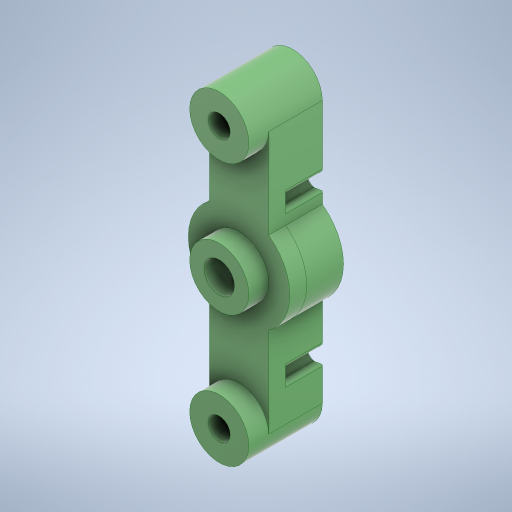
# Autodesk Inventor part: DualPMTController.MidSpacer
Saved by Autodesk Inventor 2023 (Build 270158000, 158)
## iProperties
Created: 2023-09-26
Part Number: DualPMTController.MidSpacer
Material: Generic
Document SubType Name: Modeling
Designer: Graeme
Density: 1 g/cm^3
Appearance: Default
Mass: 1.63627 g
Surface Area: 17.3966 cm^2
Volume: 1.63627 cm^3
Author: Graeme
Autodesk Inventor part; units mm, degrees
sketch "Sketch1" plane through (0, 0, 0) normal (0, 0, 1) x (1, 0, 0)
  circle A0 centre (0, 15.5) radius 1.55 projected
  circle A1 centre (0, 15.5) radius 3.5
  circle A2 centre (0, -15.5) radius 1.55 projected
  circle A3 centre (0, -15.5) radius 3.5
  circle A4 centre (0, 15.5) radius 1.3
  circle A5 centre (0, -15.5) radius 1.3
  point P0 (0, 0)
  dimension "d0" = 7
  dimension "d1" = 7
  dimension "d29" = 2.6
  dimension "d30" = 2.6
  constraints: 4 centre point, 4 coincident
  measures "d0" diameter of A1
  measures "d1" diameter of A3
  measures "d29" diameter of A4
  measures "d30" diameter of A5
ref_plane "Work Plane1" through (-88.8, 12.7, 8.6873) normal (0, 0, 1) x (1, 0, 0)
extrude "Extrusion1" add sketch "Sketch1" along normal up to surface (8.6873 mm away) contours A0 | A1 | A2 | A3
ref_plane "Work Plane2" through (0, 15.5, 4.3437) normal (0, 0, 1) x (1, 0, 0)
sketch "Sketch2" plane through (0, 15.5, 4.3437) normal (0, 0, 1) x (1, 0, 0)
  circle A0 centre (0, 0) radius 3.5 projected
  circle A1 centre (0, -31) radius 3.5 projected
  line L0 (3, -18.2) -> (3, -16.5) projected
  line L1 (3, -16.5) -> (2.8, -16.5) projected
  line L2 (2.8, -14.5) -> (2.8, -16.5) projected
  line L3 (3, -14.5) -> (2.8, -14.5) projected
  line L4 (3, -14.5) -> (3, -12.8) projected
  arc A2 (3, -12.8) -> (2.7, -12.5) centre (2.7, -12.8) ccw projected
  line L5 (2.7, -12.5) -> (1, -12.5) projected
  line L6 (1, -12.5) -> (1, -12.7) projected
  line L7 (-1, -12.7) -> (1, -12.7) projected
  line L8 (-1, -12.5) -> (-1, -12.7) projected
  line L9 (-1, -12.5) -> (-2.7, -12.5) projected
  arc A3 (-2.7, -12.5) -> (-3, -12.8) centre (-2.7, -12.8) ccw projected
  line L10 (-3, -12.8) -> (-3, -14.5) projected
  line L11 (-3, -14.5) -> (-2.8, -14.5) projected
  line L12 (-2.8, -16.5) -> (-2.8, -14.5) projected
  line L13 (-3, -16.5) -> (-2.8, -16.5) projected
  line L14 (-3, -16.5) -> (-3, -18.2) projected
  arc A4 (-3, -18.2) -> (-2.7, -18.5) centre (-2.7, -18.2) ccw projected
  line L15 (-2.7, -18.5) -> (-1, -18.5) projected
  line L16 (-1, -18.5) -> (-1, -18.3) projected
  line L17 (1, -18.3) -> (-1, -18.3) projected
  line L18 (1, -18.5) -> (1, -18.3) projected
  line L19 (1, -18.5) -> (2.7, -18.5) projected
  arc A5 (2.7, -18.5) -> (3, -18.2) centre (2.7, -18.2) ccw projected
  circle A6 centre (0, -15.5) radius 1.75 projected
  circle A7 centre (1.65, -13.85) radius 0.35 projected
  circle A8 centre (-1.65, -13.85) radius 0.35 projected
  circle A9 centre (-1.65, -17.15) radius 0.35 projected
  circle A10 centre (1.65, -17.15) radius 0.35 projected
  circle A11 centre (0, 0) radius 3.5 projected
  line L20 (-3.5, 0) -> (3.5, 0)
  line L21 (3.5, 0) -> (3.5, -31)
  line L22 (3.5, -31) -> (-3.5, -31)
  line L23 (-3.5, -31) -> (-3.5, 0)
  line L24 (0.8, -12.3) -> (2.7, -12.3)
  arc A12 (3.2, -12.8) -> (2.7, -12.3) centre (2.7, -12.8) ccw
  line L25 (3.2, -12.8) -> (3.2, -14.7)
  line L26 (3.2, -14.7) -> (3, -14.7)
  line L27 (3, -14.7) -> (3, -16.3)
  line L28 (3, -16.3) -> (3.2, -16.3)
  line L29 (3.2, -16.3) -> (3.2, -18.2)
  arc A13 (2.7, -18.7) -> (3.2, -18.2) centre (2.7, -18.2) ccw
  line L30 (2.7, -18.7) -> (0.8, -18.7)
  line L31 (0.8, -18.7) -> (0.8, -18.5)
  line L32 (0.8, -18.5) -> (-0.8, -18.5)
  line L33 (-0.8, -18.5) -> (-0.8, -18.7)
  line L34 (-0.8, -18.7) -> (-2.7, -18.7)
  arc A14 (-3.2, -18.2) -> (-2.7, -18.7) centre (-2.7, -18.2) ccw
  line L35 (-3.2, -18.2) -> (-3.2, -16.3)
  line L36 (-3.2, -16.3) -> (-3, -16.3)
  line L37 (-3, -16.3) -> (-3, -14.7)
  line L38 (-3, -14.7) -> (-3.2, -14.7)
  line L39 (-3.2, -14.7) -> (-3.2, -12.8)
  arc A15 (-2.7, -12.3) -> (-3.2, -12.8) centre (-2.7, -12.8) ccw
  line L40 (-2.7, -12.3) -> (-0.8, -12.3)
  line L41 (-0.8, -12.3) -> (-0.8, -12.5)
  line L42 (-0.8, -12.5) -> (0.8, -12.5)
  line L43 (0.8, -12.5) -> (0.8, -12.3)
  circle A16 centre (0, -15.5) radius 6
  line L44 (4.5, -12.9) -> (4.5, -13.6) projected
  line L45 (4.5, -12.9) -> (3.4823, -12.9) projected
  line L46 (3.4823, -12.9) -> (3.4823, -13.6) projected
  line L47 (4.5, -13.6) -> (3.4823, -13.6) projected
  line L48 (-3.4823, -12.9) -> (-3.4823, -13.6) projected
  line L49 (-3.4823, -12.9) -> (-4.5, -12.9) projected
  line L50 (-4.5, -12.9) -> (-4.5, -13.6) projected
  line L51 (-3.4823, -13.6) -> (-4.5, -13.6) projected
  line L52 (-4.5, -17.4) -> (-4.5, -18.1) projected
  line L53 (-3.4823, -18.1) -> (-4.5, -18.1) projected
  line L54 (-3.4823, -17.4) -> (-3.4823, -18.1) projected
  line L55 (-3.4823, -17.4) -> (-4.5, -17.4) projected
  line L56 (-0.715, -20.39) -> (0.715, -20.39) projected
  arc A17 (0.715, -20.39) -> (0.79, -20.315) centre (0.715, -20.315) ccw projected
  line L57 (0.79, -20.315) -> (0.79, -19.685) projected
  arc A18 (0.79, -19.685) -> (0.715, -19.61) centre (0.715, -19.685) ccw projected
  line L58 (0.715, -19.61) -> (-0.715, -19.61) projected
  arc A19 (-0.715, -19.61) -> (-0.79, -19.685) centre (-0.715, -19.685) ccw projected
  line L59 (-0.79, -19.685) -> (-0.79, -20.315) projected
  arc A20 (-0.79, -20.315) -> (-0.715, -20.39) centre (-0.715, -20.315) ccw projected
  arc A21 (1.29, -19.685) -> (0.715, -19.11) centre (0.715, -19.685) ccw
  line L60 (1.29, -19.685) -> (1.29, -20.315)
  arc A22 (0.715, -20.89) -> (1.29, -20.315) centre (0.715, -20.315) ccw
  line L61 (0.715, -20.89) -> (-0.715, -20.89)
  arc A23 (-1.29, -20.315) -> (-0.715, -20.89) centre (-0.715, -20.315) ccw
  line L62 (-1.29, -20.315) -> (-1.29, -19.685)
  arc A24 (-0.715, -19.11) -> (-1.29, -19.685) centre (-0.715, -19.685) ccw
  line L63 (-0.715, -19.11) -> (0.715, -19.11)
  line L64 (3.4823, -17.4) -> (3.4823, -18.1) projected
  line L65 (4.5, -18.1) -> (3.4823, -18.1) projected
  line L66 (4.5, -17.4) -> (4.5, -18.1) projected
  line L67 (4.5, -17.4) -> (3.4823, -17.4) projected
  line L68 (3.0823, -17) -> (3.0823, -18.5)
  line L69 (3.0823, -18.5) -> (4.9, -18.5)
  line L70 (4.9, -18.5) -> (4.9, -17)
  line L71 (4.9, -17) -> (3.0823, -17)
  line L72 (3.0823, -14) -> (3.0823, -12.5)
  line L73 (3.0823, -12.5) -> (4.9, -12.5)
  line L74 (4.9, -12.5) -> (4.9, -14)
  line L75 (4.9, -14) -> (3.0823, -14)
  line L76 (-4.9, -14) -> (-4.9, -12.5)
  line L77 (-4.9, -12.5) -> (-3.0823, -12.5)
  line L78 (-3.0823, -12.5) -> (-3.0823, -14)
  line L79 (-3.0823, -14) -> (-4.9, -14)
  line L80 (-4.9, -17) -> (-4.9, -18.5)
  line L81 (-4.9, -18.5) -> (-3.0823, -18.5)
  line L82 (-3.0823, -18.5) -> (-3.0823, -17)
  line L83 (-3.0823, -17) -> (-4.9, -17)
  circle A25 centre (2.83, -26) radius 0.52
  circle A26 centre (0.29, -26) radius 0.52
  circle A27 centre (-2.25, -26) radius 0.52
  circle A28 centre (2.83, -8.22) radius 0.52
  circle A29 centre (0.29, -8.22) radius 0.52
  circle A30 centre (-2.25, -8.22) radius 0.52
  circle A31 centre (2.83, -8.22) radius 0.72
  circle A32 centre (0.29, -8.22) radius 0.72
  circle A33 centre (-2.25, -8.22) radius 0.72
  circle A34 centre (2.83, -26) radius 0.72
  circle A35 centre (0.29, -26) radius 0.72
  circle A36 centre (-2.25, -26) radius 0.72
  line L84 (-0.8, -18.7) -> (0.8, -18.7)
  line L85 (-0.8, -12.3) -> (0.8, -12.3)
  point P0 (0, -15.5)
  point P1 (-3.5, -17)
  point P2 (-3.5, -14)
  point P3 (-3.1, -12.5)
  point P4 (3.1, -12.5)
  point P5 (3.5, -14)
  point P6 (3.5, -17)
  point P7 (3.1, -18.5)
  point P8 (-3.1, -18.5)
  point P9 (3.5, -10.6266)
  point P10 (-3.5, -10.6266)
  point P11 (-3.5, -20.3734)
  point P12 (3.5, -20.3734)
  point P13 (3.5, -8.4836)
  point P14 (3.5, -7.9564)
  point P15 (3.5, -26.2636)
  point P16 (3.5, -25.7364)
  dimension "d4" = 0.2
  dimension "d5" = 12
  dimension "d6" = 0.5
  dimension "d7" = 0.4
  dimension "d8" = 0.4
  dimension "d9" = 0.4
  dimension "d10" = 0.4
  dimension "d13" = 0.2
  dimension "d14" = 0.2
  dimension "d15" = 0.2
  dimension "d16" = 0.2
  dimension "d17" = 0.2
  dimension "d18" = 0.2
  constraints: 92 end point, 21 centre point, 16 point on circle, 3 parallel, 2 horizontal, 2 tangent, 1 coincident, 1 horizontal alignment, 1 perpendicular, 57 other
  measures "d4" distance between parallel lines of L5 L24
  measures "d5" diameter of A16
  measures "d6" radial gap between concentric circles of A18 A21
  measures "d7" distance between parallel lines of L67 L71
  measures "d8" distance between parallel lines of L47 L75
  measures "d9" distance between parallel lines of L51 L79
  measures "d10" distance between parallel lines of L55 L83
  measures "d13" radial gap between concentric circles of A28 A31
  measures "d14" radial gap between concentric circles of A29 A32
  measures "d15" radial gap between concentric circles of A30 A33
  measures "d16" radial gap between concentric circles of A25 A34
  measures "d17" radial gap between concentric circles of A26 A35
  measures "d18" radial gap between concentric circles of A27 A36
ref_plane "Work Plane3" through (-89.5, -19, 0) normal (0, 0, 1) x (1, 0, 0)
extrude "Extrusion2" add sketch "Sketch2" against normal up to surface (4.3437 mm away) contours L21 A31 A16 L23 A0 | A16 L21 L73 A12 L24 L85 L40 A15 L77 L23 | L23 L77 L76 L79 L83 L80 L81 A16 | A16 L21 L69 L70 L71 L75 L74 L73 | A16 L21 A34 A1 L23 | L23 L81 A14 L34 L84 L30 A13 L69 L21 A16
sketch "Sketch3" plane through (0, 15.5, 4.3437) normal (0, 0, 1) x (1, 0, 0)
  arc A0 (-3.5, 0) -> (3.5, 0) centre (0, 0) ccw projected
  arc A1 (3.5, -31) -> (-3.5, -31) centre (0, -31) ccw projected
  line L0 (-3.5, 0) -> (3.5, 0)
  line L1 (3.5, 0) -> (3.5, -31)
  line L2 (3.5, -31) -> (-3.5, -31)
  line L3 (-3.5, -31) -> (-3.5, 0)
  circle A2 centre (0, -15.5) radius 6
  arc A3 (-3.5, -10.6266) -> (-3.5, -20.3734) centre (0, -15.5) ccw projected
  circle A4 centre (0, -15.5) radius 1.55 projected
  circle A5 centre (0, -15.5) radius 1.8
  point P0 (-3.5, -10.6266)
  point P1 (-3.5, -20.3734)
  point P2 (3.5, -20.3734)
  point P3 (3.5, -10.6266)
  dimension "d24" = 3.6
  constraints: 8 end point, 2 centre point, 2 coincident, 2 parallel, 2 point on circle, 1 equal radius, 1 horizontal, 1 perpendicular
  measures "d24" diameter of A5
extrude "Extrusion3" add sketch "Sketch3" along normal blind 2 contours A0 L1 A2 L3 | A2 L1 L3 | L3 A2 | A2 L1 | A2 L1 A1 L3
chamfer "Chamfer1" distance 0.5 angle 45 6 edges at (2.11, -10.5, 0) (-0.43, -10.5, 0) (-2.97, -10.5, 0) (2.11, 7.28, 0) (-0.43, 7.28, 0) (-2.97, 7.28, 0)
sketch "Sketch4" plane through (0, 15.5, 6.3437) normal (0, 0, 1) x (1, 0, 0)
  circle A0 centre (0, -15.5) radius 1.8 projected
  circle A1 centre (0, -15.5) radius 3.5
  point P0 (0, -15.5)
  dimension "d25" = 7
  constraints: 1 centre point, 1 coincident
  measures "d25" diameter of A1
extrude "Extrusion4" add sketch "Sketch4" along normal up to surface (2.3437 mm away)
fillet "Fillet1" radius 0.5 4 edges at (3.5, -10.2364, 2.4218) (3.5, -10.7636, 2.4218) (3.5, 7.0164, 2.4218) (3.5, 7.5436, 2.4218)
equation "\"d1\" = d0"
body "Solid1"
